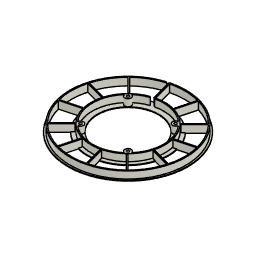
ringclock_center (Autodesk Fusion 360 design; units mm, degrees)
Autodesk Fusion 360 part; units mm, degrees
sketch "Skizze1" plane through (0, 0, 0) normal (0, 0, 1) x (1, 0, 0)
  circle A0 centre (0, 0) radius 103
  dimension "d1" = 206
  constraint coincident A0.centre origin
  measures "d1" diameter of A0
extrude "Extrusion1" add sketch "Skizze1" along normal blind 1
sketch "Skizze2" plane through (0, 0, 1) normal (0, 0, 1) x (-1, 0, 0)
  circle A0 centre (0, 0) radius 103
  circle A1 centre (0, 0) radius 100
  circle A2 centre (0, 0) radius 98
  dimension "d4" = 200
  dimension "d5" = 196
  constraint coincident A0.centre A1.centre
  measures "d4" diameter of A1
  measures "d5" diameter of A2
extrude "Extrusion2" add sketch "Skizze2" along normal blind 12 contours A1
sketch "Skizze5" plane through (0, 0, 1) normal (0, 0, 1) x (-1, 0, 0)
  circle A0 centre (0, 0) radius 98
  circle A1 centre (0, 0) radius 63.5
  circle A2 centre (0, 0) radius 61.5
  line L0 (-25.3643, -94.6607) -> (-16.435, -61.3363)
  line L1 (-27.2908, -94.1234) -> (-18.3587, -60.7882)
  line L2 (0, 0) -> (0, -37) construction
  line L3 (25.3643, -94.6607) -> (16.435, -61.3363)
  line L4 (23.4271, -95.1587) -> (14.495, -61.8235)
  line L5 (69.2965, -69.2965) -> (44.9013, -44.9013)
  line L6 (67.8678, -70.6962) -> (43.4648, -46.2932)
  line L7 (94.6607, -25.3643) -> (61.3363, -16.435)
  line L8 (94.1234, -27.2908) -> (60.7882, -18.3587)
  line L9 (94.6607, 25.3643) -> (61.3363, 16.435)
  line L10 (95.1587, 23.4271) -> (61.8235, 14.495)
  line L11 (69.2965, 69.2965) -> (44.9013, 44.9013)
  line L12 (70.6962, 67.8678) -> (46.2932, 43.4648)
  line L13 (25.3643, 94.6607) -> (16.435, 61.3363)
  line L14 (27.2908, 94.1234) -> (18.3587, 60.7882)
  line L15 (-25.3643, 94.6607) -> (-16.435, 61.3363)
  line L16 (-23.4271, 95.1587) -> (-14.495, 61.8235)
  line L17 (-69.2965, 69.2965) -> (-44.9013, 44.9013)
  line L18 (-67.8678, 70.6962) -> (-43.4648, 46.2932)
  line L19 (-94.6607, 25.3643) -> (-61.3363, 16.435)
  line L20 (-94.1234, 27.2908) -> (-60.7882, 18.3587)
  line L21 (-94.6607, -25.3643) -> (-61.3363, -16.435)
  line L22 (-95.1587, -23.4271) -> (-61.8235, -14.495)
  line L23 (-69.2965, -69.2965) -> (-44.9013, -44.9013)
  line L24 (-70.6962, -67.8678) -> (-46.2932, -43.4648)
  dimension "d53" = 127
  dimension "d54" = 123
  dimension "d55" = 2
  dimension "d56" = 15
  dimension "d58" = 360
  constraint coincident A0.centre A1.centre
  constraint coincident A0 L0.start
  constraint coincident A1 L0.end
  constraint coincident A0 L1.start
  constraint coincident A1 L1.end
  constraint parallel L0 L1
  constraint coincident A0.centre L0
  constraint vertical L2
  measures "d53" diameter of A1
  measures "d54" diameter of A2
  measures "d55" distance of L0 L1
  measures "d56" angle of L0 L2
extrude "Extrusion4" add sketch "Skizze5" along normal blind 12 contours A0 A1 L9 L10 | A0 A1 L7 L8 | A1 | A0 A1 L11 L12 | A0 A1 L5 L6 | A0 A1 L13 L14 | A0 A1 L3 L4 | A0 A1 L15 L16 | A0 A1 L0 L1 | A0 A1 L17 L18 | A0 A1 L23 L24 | A0 A1 L19 L20 | A0 A1 L21 L22
extrude "Extrusion8" cut 12 faces at (-16.4083, 84.7761, 1) (28.178, 81.6224, 1) (65.2141, 56.5981, 1) (84.7761, 16.4083, 1) (81.6224, -28.178, 1) (56.5981, -65.2141, 1) (16.4083, -84.7761, 1) (-28.178, -81.6224, 1) (-65.2141, -56.5981, 1) (-84.7761, -16.4083, 1) (-81.6224, 28.178, 1) (-56.5981, 65.2141, 1) along direction (0, 0, -1) blind 10
sketch "Skizze6" plane through (0, 0, 13) normal (0, 0, 1) x (-1, 0, 0)
  arc A0 (69.2965, 69.2965) -> (27.2908, 94.1234) centre (0, 0) ccw
  line L0 (69.2965, 69.2965) -> (44.9013, 44.9013)
  arc A1 (44.9013, 44.9013) -> (18.3587, 60.7882) centre (0, 0) ccw
  line L1 (18.3587, 60.7882) -> (27.2908, 94.1234)
  line L2 (25.3643, 94.6607) -> (16.435, 61.3363)
  arc A2 (16.435, 61.3363) -> (-14.495, 61.8235) centre (0, 0) ccw
  line L3 (-14.495, 61.8235) -> (-23.4271, 95.1587)
  line L4 (94.6607, 25.3643) -> (61.3363, 16.435)
  arc A3 (61.3363, 16.435) -> (46.2932, 43.4648) centre (0, 0) ccw
  line L5 (46.2932, 43.4648) -> (70.6962, 67.8678)
  line L6 (-25.3643, 94.6607) -> (-16.435, 61.3363)
  arc A4 (-16.435, 61.3363) -> (-43.4648, 46.2932) centre (0, 0) ccw
  line L7 (-43.4648, 46.2932) -> (-67.8678, 70.6962)
  line L8 (94.6607, -25.3643) -> (61.3363, -16.435)
  arc A5 (61.3363, -16.435) -> (61.8235, 14.495) centre (0, 0) ccw
  line L9 (61.8235, 14.495) -> (95.1587, 23.4271)
  line L10 (-69.2965, 69.2965) -> (-44.9013, 44.9013)
  arc A6 (-44.9013, 44.9013) -> (-60.7882, 18.3587) centre (0, 0) ccw
  line L11 (-60.7882, 18.3587) -> (-94.1234, 27.2908)
  line L12 (69.2965, -69.2965) -> (44.9013, -44.9013)
  arc A7 (44.9013, -44.9013) -> (60.7882, -18.3587) centre (0, 0) ccw
  line L13 (60.7882, -18.3587) -> (94.1234, -27.2908)
  line L14 (-94.6607, 25.3643) -> (-61.3363, 16.435)
  arc A8 (-61.3363, 16.435) -> (-61.8235, -14.495) centre (0, 0) ccw
  line L15 (-61.8235, -14.495) -> (-95.1587, -23.4271)
  line L16 (25.3643, -94.6607) -> (16.435, -61.3363)
  arc A9 (16.435, -61.3363) -> (43.4648, -46.2932) centre (0, 0) ccw
  line L17 (43.4648, -46.2932) -> (67.8678, -70.6962)
  line L18 (-94.6607, -25.3643) -> (-61.3363, -16.435)
  arc A10 (-61.3363, -16.435) -> (-46.2932, -43.4648) centre (0, 0) ccw
  line L19 (-46.2932, -43.4648) -> (-70.6962, -67.8678)
  line L20 (-25.3643, -94.6607) -> (-16.435, -61.3363)
  arc A11 (-16.435, -61.3363) -> (14.495, -61.8235) centre (0, 0) ccw
  line L21 (14.495, -61.8235) -> (23.4271, -95.1587)
  circle A12 centre (0, 0) radius 61.5
  line L22 (-69.2965, -69.2965) -> (-44.9013, -44.9013)
  arc A13 (-44.9013, -44.9013) -> (-18.3587, -60.7882) centre (0, 0) ccw
  line L23 (-18.3587, -60.7882) -> (-27.2908, -94.1234)
  circle A14 centre (0, 0) radius 100
  circle A15 centre (0, 0) radius 64.5
  circle A16 centre (0, 0) radius 63.5
  arc A17 (25.3643, 94.6607) -> (-23.4271, 95.1587) centre (0, 0) ccw
  arc A18 (94.6607, 25.3643) -> (70.6962, 67.8678) centre (0, 0) ccw
  arc A19 (-25.3643, 94.6607) -> (-67.8678, 70.6962) centre (0, 0) ccw
  arc A20 (94.6607, -25.3643) -> (95.1587, 23.4271) centre (0, 0) ccw
  arc A21 (-69.2965, 69.2965) -> (-94.1234, 27.2908) centre (0, 0) ccw
  arc A22 (69.2965, -69.2965) -> (94.1234, -27.2908) centre (0, 0) ccw
  arc A23 (-94.6607, 25.3643) -> (-95.1587, -23.4271) centre (0, 0) ccw
  arc A24 (25.3643, -94.6607) -> (67.8678, -70.6962) centre (0, 0) ccw
  arc A25 (-94.6607, -25.3643) -> (-70.6962, -67.8678) centre (0, 0) ccw
  arc A26 (-25.3643, -94.6607) -> (23.4271, -95.1587) centre (0, 0) ccw
  arc A27 (-69.2965, -69.2965) -> (-27.2908, -94.1234) centre (0, 0) ccw
  dimension "d61" = 127
  dimension "d62" = 129
  constraint concentric A0 A15
  constraint coincident A0.centre A1.centre
  measures "d61" diameter of A16
  measures "d62" diameter of A15
extrude "Extrusion5" cut sketch "Skizze6" against normal blind 12 contours L0 L5 A15 A16 | L1 L2 A15 A16 | L4 L9 A15 A16 | L3 L6 A15 A16 | L7 L10 A15 A16 | L8 L13 A15 A16 | L11 L14 A15 A16 | L12 L17 A15 A16 | L15 L18 A15 A16 | L16 L21 A15 A16 | L19 L22 A15 A16 | L20 L23 A15 A16
extrude "Extrusion10" add 1 faces at (-14.7974, 62.0938, 1) along direction (0, 0, 1) blind 12
sketch "Skizze7" plane through (0, 0, 13) normal (0, 0, 1) x (-1, 0, 0)
  circle A0 centre (0, 0) radius 100
  arc A1 (62.7899, 14.7539) -> (62.3022, 16.6938) centre (0, 0) ccw
  line L0 (62.7899, 14.7539) -> (95.1587, 23.4271)
  arc A2 (-69.2965, -69.2965) -> (-27.2908, -94.1234) centre (0, 0) ccw
  line L1 (94.6607, -25.3643) -> (62.3022, -16.6938)
  arc A3 (61.7546, -18.6177) -> (62.3022, -16.6938) centre (0, 0) ccw
  line L2 (61.7546, -18.6177) -> (94.1234, -27.2908)
  line L3 (69.2965, -69.2965) -> (45.6084, -45.6084)
  arc A4 (44.1722, -47.0007) -> (45.6084, -45.6084) centre (0, 0) ccw
  line L4 (44.1722, -47.0007) -> (67.8678, -70.6962)
  line L5 (25.3643, -94.6607) -> (16.435, -61.3363)
  line L6 (14.495, -61.8235) -> (23.4271, -95.1587)
  line L7 (-25.3643, -94.6607) -> (-16.6938, -62.3022)
  line L8 (-18.6177, -61.7546) -> (-27.2908, -94.1234)
  line L9 (-69.2965, -69.2965) -> (-45.6084, -45.6084)
  arc A5 (-47.0007, -44.1722) -> (-45.6084, -45.6084) centre (0, 0) ccw
  line L10 (-47.0007, -44.1722) -> (-70.6962, -67.8678)
  line L11 (-94.6607, -25.3643) -> (-62.3022, -16.6938)
  arc A6 (-62.7899, -14.7539) -> (-62.3022, -16.6938) centre (0, 0) ccw
  line L12 (-62.7899, -14.7539) -> (-95.1587, -23.4271)
  line L13 (-94.6607, 25.3643) -> (-62.3022, 16.6938)
  arc A7 (-61.7546, 18.6177) -> (-62.3022, 16.6938) centre (0, 0) ccw
  line L14 (-61.7546, 18.6177) -> (-94.1234, 27.2908)
  line L15 (-69.2965, 69.2965) -> (-45.6084, 45.6084)
  arc A8 (-44.1722, 47.0007) -> (-45.6084, 45.6084) centre (0, 0) ccw
  line L16 (-44.1722, 47.0007) -> (-67.8678, 70.6962)
  line L17 (-25.3643, 94.6607) -> (-16.6938, 62.3022)
  arc A9 (-14.7539, 62.7899) -> (-16.6938, 62.3022) centre (0, 0) ccw
  line L18 (-14.7539, 62.7899) -> (-23.4271, 95.1587)
  line L19 (25.3643, 94.6607) -> (16.6938, 62.3022)
  arc A10 (18.6177, 61.7546) -> (16.6938, 62.3022) centre (0, 0) ccw
  line L20 (18.6177, 61.7546) -> (27.2908, 94.1234)
  line L21 (69.2965, 69.2965) -> (45.6084, 45.6084)
  arc A11 (47.0007, 44.1722) -> (45.6084, 45.6084) centre (0, 0) ccw
  line L22 (47.0007, 44.1722) -> (70.6962, 67.8678)
  line L23 (94.6607, 25.3643) -> (62.3022, 16.6938)
  line L24 (16.435, -61.3363) -> (24.5878, -91.763)
  line L25 (24.5878, -91.763) -> (26.5197, -91.2453)
  line L26 (26.5197, -91.2453) -> (28.5902, -98.9727)
  line L27 (28.5902, -98.9727) -> (26.6584, -99.4904)
  line L28 (26.6584, -99.4904) -> (25.3643, -94.6607)
  arc A12 (-25.3643, -94.6607) -> (23.4271, -95.1587) centre (0, 0) ccw
  arc A13 (-18.6177, -61.7546) -> (-16.6938, -62.3022) centre (0, 0) ccw
  arc A14 (16.435, -61.3363) -> (14.495, -61.8235) centre (0, 0) ccw
  arc A15 (-94.6607, -25.3643) -> (-70.6962, -67.8678) centre (0, 0) ccw
  arc A16 (-94.6607, 25.3643) -> (-95.1587, -23.4271) centre (0, 0) ccw
  arc A17 (-69.2965, 69.2965) -> (-94.1234, 27.2908) centre (0, 0) ccw
  arc A18 (-25.3643, 94.6607) -> (-67.8678, 70.6962) centre (0, 0) ccw
  arc A19 (25.3643, 94.6607) -> (-23.4271, 95.1587) centre (0, 0) ccw
  arc A20 (69.2965, 69.2965) -> (27.2908, 94.1234) centre (0, 0) ccw
  arc A21 (94.6607, 25.3643) -> (70.6962, 67.8678) centre (0, 0) ccw
  arc A22 (94.6607, -25.3643) -> (95.1587, 23.4271) centre (0, 0) ccw
  arc A23 (69.2965, -69.2965) -> (94.1234, -27.2908) centre (0, 0) ccw
  arc A24 (25.3643, -94.6607) -> (67.8678, -70.6962) centre (0, 0) ccw
  circle A25 centre (0, 0) radius 61.5
  line L29 (17.4703, -65.2) -> (21.334, -64.1647)
  line L30 (21.334, -64.1647) -> (19.2634, -56.4373)
  line L31 (19.2634, -56.4373) -> (15.3997, -57.4726)
  line L32 (15.3997, -57.4726) -> (17.4703, -65.2)
  dimension "d65" = 2
  dimension "d66" = 5
  dimension "d100" = 8
  dimension "d101" = 8
  dimension "d102" = 4
  dimension "d103" = 4
  constraint coincident L5.end L24.start
  constraint parallel L5 L24
  constraint perpendicular L5 L25
  constraint perpendicular L25 L26
  constraint perpendicular L26 L27
  constraint coincident L5.start L28.end
  constraint parallel L26 L28
  constraint coincident L24 L29.start
  constraint perpendicular L24 L29
  constraint perpendicular L29 L30
  constraint perpendicular L30 L31
  constraint collinear L24 L32
  measures "d65" distance of L5 L26
  measures "d66" distance of L27 L5.start
  measures "d100" distance of L25 L27
  measures "d101" distance of L29 L31
  measures "d102" distance of L30 L32
  measures "d103" distance of L5.end L31
extrude "Extrusion6" cut sketch "Skizze7" against normal blind 12 contours A0 L26 L28 A24 | A0 L26 L27 L28 | L5 L25 L26 A24 | L5 L24 A14 L29 L30 L32 | A14 A25 L30 L32 | A25 L30 L31 L32 picked at (17.7141, -57.5227)
fillet "Abrundung1" radius 3 1 edges at (-27.8086, 96.0556, 7)
fillet "Abrundung2" radius 2 1 edges at (-20.2661, 60.1792, 7)
fillet "Abrundung3" radius 2 1 edges at (-15.9174, 59.4044, 7)
sketch "Skizze8" plane through (0, 0, 1) normal (0, 0, 1) x (-1, 0, 0)
  circle A0 centre (0, 0) radius 103
  arc A1 (30.622, -95.1961) -> (25.8819, -96.5926) centre (0, 0) ccw
  arc A2 (27.2908, -94.1234) -> (30.622, -95.1961) centre (29.7034, -92.3402) ccw
  arc A3 (25.3643, -94.6607) -> (27.2908, -94.1234) centre (0, 0) ccw
  circle A4 centre (41, -41) radius 2.25
  circle A5 centre (41, -41) radius 5.5
  circle A6 centre (-41, -41) radius 2.25
  circle A7 centre (-41, -41) radius 5.5
  circle A8 centre (41, 41) radius 2.25
  circle A9 centre (41, 41) radius 5.5
  circle A10 centre (-41, 41) radius 2.25
  circle A11 centre (-41, 41) radius 5.5
  line L0 (25.3643, -94.6607) -> (25.8819, -96.5926)
  dimension "d78" = 41
  dimension "d79" = 41
  dimension "d80" = 4.5
  dimension "d81" = 11
  dimension "d84" = -82
  dimension "d85" = 82
  constraint concentric A4 A5
  measures "d78" horizontal distance of A0.centre A4.centre
  measures "d79" vertical distance of A0.centre A4.centre
  measures "d80" diameter of A4
  measures "d81" diameter of A5
extrude "Extrusion7" add sketch "Skizze8" along normal blind 12 contours A5 | A7 | A9 | A11
sketch "Skizze9" plane through (0, 0, 1) normal (0, 0, 1) x (-1, 0, 0)
  arc A0 (46.4554, -40.3007) -> (40.3007, -46.4554) centre (41, -41) ccw
  arc A1 (46.4554, -40.3007) -> (46.4554, 40.3007) centre (0, 0) ccw
  arc A2 (40.3007, 46.4554) -> (46.4554, 40.3007) centre (41, 41) ccw
  arc A3 (40.3007, 46.4554) -> (-40.3007, 46.4554) centre (0, 0) ccw
  arc A4 (-46.4554, 40.3007) -> (-40.3007, 46.4554) centre (-41, 41) ccw
  arc A5 (-46.4554, 40.3007) -> (-46.4554, -40.3007) centre (0, 0) ccw
  arc A6 (-40.3007, -46.4554) -> (-46.4554, -40.3007) centre (-41, -41) ccw
  arc A7 (-40.3007, -46.4554) -> (14.0385, -59.8763) centre (0, 0) ccw
  arc A8 (16.4269, -61.3059) -> (14.0385, -59.8763) centre (14.495, -61.8235) ccw
  line L0 (16.4269, -61.3059) -> (16.435, -61.3363)
  arc A9 (16.435, -61.3363) -> (22.3342, -59.4427) centre (0, 0) ccw
  circle A10 centre (0, 0) radius 52.5
  arc A11 (19.7474, -58.2434) -> (22.3342, -59.4427) centre (21.6308, -57.5705) ccw
  arc A12 (19.7474, -58.2434) -> (40.3007, -46.4554) centre (0, 0) ccw
  dimension "d94" = 105
  constraint concentric A1 A10
  measures "d94" diameter of A10
extrude "Extrusion11" cut sketch "Skizze9" against normal blind 10 contours A0 A2 A4 A6 A10
sketch "Skizze10" plane through (0, 0, 0) normal (0, 0, -1) x (1, 0, 0)
  arc A0 (-36.8291, -37.4148) -> (-37.4148, -36.8291) centre (-41, -41) ccw
  arc A1 (-37.4148, 36.8291) -> (-37.4148, -36.8291) centre (0, 0) ccw
  arc A2 (-37.4148, 36.8291) -> (-36.8291, 37.4148) centre (-41, 41) ccw
  arc A3 (36.8291, 37.4148) -> (-36.8291, 37.4148) centre (0, 0) ccw
  arc A4 (36.8291, 37.4148) -> (37.4148, 36.8291) centre (41, 41) ccw
  arc A5 (37.4148, -36.8291) -> (37.4148, 36.8291) centre (0, 0) ccw
  arc A6 (37.4148, -36.8291) -> (36.8291, -37.4148) centre (41, -41) ccw
  arc A7 (-36.8291, -37.4148) -> (36.8291, -37.4148) centre (0, 0) ccw
  arc A8 (-60.7882, -18.3587) -> (-44.9013, -44.9013) centre (0, 0) ccw
  line L0 (-44.9013, -44.9013) -> (-69.2965, -69.2965)
  arc A9 (-94.1234, -27.2908) -> (-69.2965, -69.2965) centre (0, 0) ccw
  line L1 (-94.1234, -27.2908) -> (-60.7882, -18.3587)
  arc A10 (-46.2932, 43.4648) -> (-61.3363, 16.435) centre (0, 0) ccw
  line L2 (-61.3363, 16.435) -> (-94.6607, 25.3643)
  arc A11 (-70.6962, 67.8678) -> (-94.6607, 25.3643) centre (0, 0) ccw
  line L3 (-70.6962, 67.8678) -> (-46.2932, 43.4648)
  arc A12 (23.4271, 95.1587) -> (-25.3643, 94.6607) centre (0, 0) ccw
  line L4 (23.4271, 95.1587) -> (14.495, 61.8235)
  arc A13 (14.495, 61.8235) -> (-16.435, 61.3363) centre (0, 0) ccw
  line L5 (-16.435, 61.3363) -> (-25.3643, 94.6607)
  arc A14 (94.1234, 27.2908) -> (69.2965, 69.2965) centre (0, 0) ccw
  line L6 (94.1234, 27.2908) -> (60.7882, 18.3587)
  arc A15 (60.7882, 18.3587) -> (44.9013, 44.9013) centre (0, 0) ccw
  line L7 (44.9013, 44.9013) -> (69.2965, 69.2965)
  arc A16 (70.6962, -67.8678) -> (94.6607, -25.3643) centre (0, 0) ccw
  line L8 (70.6962, -67.8678) -> (46.2932, -43.4648)
  arc A17 (46.2932, -43.4648) -> (61.3363, -16.435) centre (0, 0) ccw
  line L9 (61.3363, -16.435) -> (94.6607, -25.3643)
  arc A18 (-14.495, -61.8235) -> (16.435, -61.3363) centre (0, 0) ccw
  line L10 (16.435, -61.3363) -> (25.3643, -94.6607)
  arc A19 (-23.4271, -95.1587) -> (25.3643, -94.6607) centre (0, 0) ccw
  line L11 (-23.4271, -95.1587) -> (-14.495, -61.8235)
  arc A20 (27.2908, -94.1234) -> (69.2965, -69.2965) centre (0, 0) ccw
  line L12 (27.2908, -94.1234) -> (18.3587, -60.7882)
  arc A21 (18.3587, -60.7882) -> (44.9013, -44.9013) centre (0, 0) ccw
  line L13 (44.9013, -44.9013) -> (69.2965, -69.2965)
  arc A22 (95.1587, -23.4271) -> (94.6607, 25.3643) centre (0, 0) ccw
  line L14 (95.1587, -23.4271) -> (61.8235, -14.495)
  arc A23 (61.8235, -14.495) -> (61.3363, 16.435) centre (0, 0) ccw
  line L15 (61.3363, 16.435) -> (94.6607, 25.3643)
  arc A24 (67.8678, 70.6962) -> (25.3643, 94.6607) centre (0, 0) ccw
  line L16 (67.8678, 70.6962) -> (43.4648, 46.2932)
  arc A25 (43.4648, 46.2932) -> (16.435, 61.3363) centre (0, 0) ccw
  line L17 (16.435, 61.3363) -> (25.3643, 94.6607)
  arc A26 (-18.3587, 60.7882) -> (-44.9013, 44.9013) centre (0, 0) ccw
  line L18 (-44.9013, 44.9013) -> (-69.2965, 69.2965)
  arc A27 (-27.2908, 94.1234) -> (-69.2965, 69.2965) centre (0, 0) ccw
  line L19 (-27.2908, 94.1234) -> (-18.3587, 60.7882)
  arc A28 (-61.8235, 14.495) -> (-61.3363, -16.435) centre (0, 0) ccw
  line L20 (-61.3363, -16.435) -> (-94.6607, -25.3643)
  arc A29 (-95.1587, 23.4271) -> (-94.6607, -25.3643) centre (0, 0) ccw
  line L21 (-95.1587, 23.4271) -> (-61.8235, 14.495)
  arc A30 (-43.4648, -46.2932) -> (-16.435, -61.3363) centre (0, 0) ccw
  line L22 (-16.435, -61.3363) -> (-25.3643, -94.6607)
  arc A31 (-67.8678, -70.6962) -> (-25.3643, -94.6607) centre (0, 0) ccw
  line L23 (-67.8678, -70.6962) -> (-43.4648, -46.2932)
  circle A32 centre (0, 0) radius 103
  circle A33 centre (0, 0) radius 70
  dimension "d97" = 140
  constraint coincident A1.centre A3.centre
  measures "d97" diameter of A33
extrude "Extrusion12" add sketch "Skizze10" against normal blind 1 contours A8 L0 L1 A33 | A28 L20 L21 A33 | A30 L22 L23 A33 | A10 L2 L3 A33 | A18 L10 L11 A33 | A26 L18 L19 A33 | L12 A21 L13 A33 | L4 A13 L5 A33 | L8 A17 L9 A33 | L16 A25 L17 A33 | L14 A23 L15 A33 | L6 A15 L7 A33
